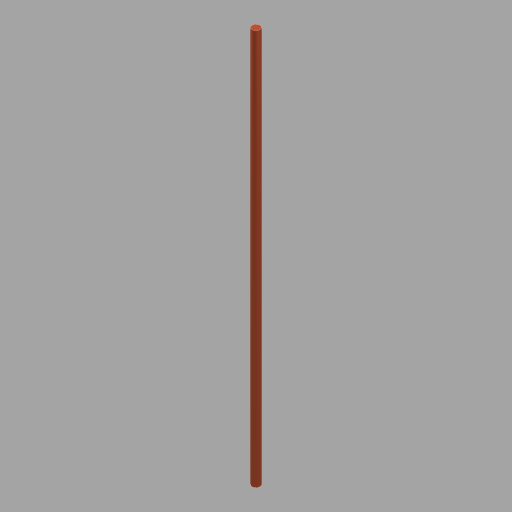
# Autodesk Inventor part: EpoxyFitThroughKF16_wire
Saved by Autodesk Inventor 2024 (Build 280153020, 153B)
## iProperties
Created: 2023-10-02
Part Number: EpoxyFitThroughKF16_wire
Material: Copper
Document SubType Name: Modeling
Designer: schanen
Density: 8.94 g/cm^3
Appearance: Copper - Satin
Author: schanen
Autodesk Inventor part; units mm, degrees
ref_plane "YZ Plane" through (0, 0, 0) normal (1, 0, 0) x (0, 1, 0)
ref_plane "XZ Plane" through (0, 0, 0) normal (0, 1, 0) x (-1, 0, 0)
ref_plane "XY Plane" through (0, 0, 0) normal (0, 0, 1) x (1, 0, 0)
sketch "Sketch1" plane through (0, 0, 0) normal (0, 0, 1) x (1, 0, 0)
  line L0 (0, 0) -> (-0.5, 0)
  line L1 (-0.5, 0) -> (-0.5, 50)
  line L2 (-0.5, 50) -> (0, 50)
  line L3 (0, 50) -> (0, 0)
  dimension "d0" = 0.5
  dimension "d1" = 50
  constraints: 8 end point, 2 parallel, 1 horizontal, 1 perpendicular
  measures "d0" distance of L1.end L2.end
  measures "d1" distance of L0.end L1.end
revolve "Revolution1" add sketch "Sketch1" angle 360 about axis through (0, 50, 0) along (0, -1, 0)
body "Solid1"
